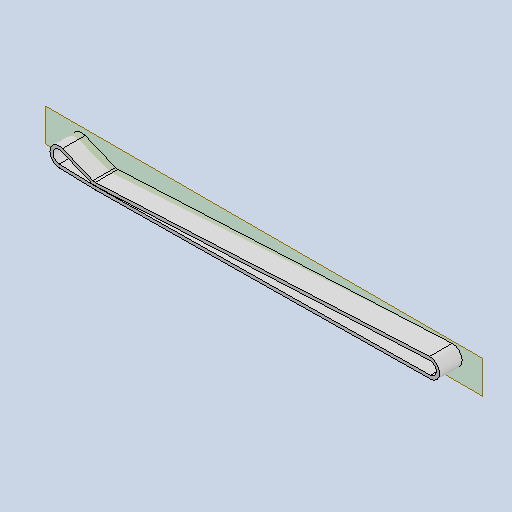
# Autodesk Inventor part: Cata rubber bands
Saved by Autodesk Inventor 2023.2 (Build 272271030, 271C)
## iProperties
Created: 2023-05-20
Part Number: Cata rubber bands
Material: Generic
Document SubType Name: Modeling
Designer: Main Account
Density: 1 g/cm^3
Appearance: Default
Author: Main Account
Autodesk Inventor part; units mm, degrees
ref_plane "YZ Plane" through (0, 0, 0) normal (1, 0, 0) x (0, 1, 0)
ref_plane "XZ Plane" through (0, 0, 0) normal (0, 1, 0) x (-1, 0, 0)
ref_plane "XY Plane" through (0, 0, 0) normal (0, 0, 1) x (1, 0, 0)
sketch "Sketch1" plane through (0, 0, 0) normal (0, 0, 1) x (1, 0, 0)
  circle A0 centre (-188.587, -221.4819) radius 3.0353 construction
  circle A1 centre (-168.9013, -220.2863) radius 3.0353 construction
  circle A2 centre (15.875, -215.9) radius 3.0353 construction
  arc A3 (-169.9939, -223.1182) -> (-168.6946, -223.3146) centre (-168.9013, -220.2863) ccw
  arc A4 (-187.3572, -218.2946) -> (-188.6171, -224.898) centre (-188.587, -221.4819) ccw
  arc A5 (-186.7273, -216.6619) -> (-188.6325, -226.648) centre (-188.587, -221.4819) ccw
  arc A6 (15.9814, -219.3146) -> (15.6425, -212.4916) centre (15.875, -215.9) ccw
  arc A7 (16.0359, -221.0638) -> (15.5233, -210.7457) centre (15.875, -215.9) ccw
  line L0 (-169.9939, -223.1182) -> (-186.7273, -216.6619)
  line L1 (-168.9589, -226.8214) -> (-188.6325, -226.648)
  line L2 (-188.6171, -224.898) -> (-168.9434, -225.0715)
  line L3 (-170.6238, -224.7509) -> (-187.3572, -218.2946)
  line L4 (-168.6946, -223.3146) -> (15.5233, -210.7457)
  line L5 (15.6425, -212.4916) -> (-168.5755, -225.0605)
  line L6 (15.9814, -219.3146) -> (-168.7523, -225.0693)
  line L7 (-168.6978, -226.8185) -> (16.0359, -221.0638)
  arc A8 (-170.6238, -224.7509) -> (-168.5755, -225.0605) centre (-168.9013, -220.2863) ccw
  arc A9 (-168.9589, -226.8214) -> (-168.6978, -226.8185) centre (-168.9013, -220.2863) ccw
  arc A10 (-164.3235, -224.9314) -> (-164.1549, -224.7589) centre (-168.9013, -220.2863) ccw
  point P0 (0, 0)
  point P1 (-192.7723, -212.6051)
  point P2 (-183.4432, -220.9999)
  point P3 (-202.7453, -212.6946)
  point P4 (-199.5727, -216.4604)
  point P5 (-186.4, -216.7421)
  dimension "d0" = 0
  dimension "d2" = 0.381
  dimension "d3" = 1.75
  dimension "d9" = 1.75
  dimension "d10" = 1.75
  dimension "d11" = 0.381
  dimension "d12" = 1.75
  constraints: 18 point on circle, 16 end point, 16 tangent, 8 centre point, 2 point on line
  measures "d0" radial gap between concentric circles of A1 A3
  measures "d2" radial gap between concentric circles of A0 A4
  measures "d3" radial gap between concentric circles of A4 A5
  measures "d9" radial gap between concentric circles of A3 A8
  measures "d10" radial gap between concentric circles of A9 A8
  measures "d11" radial gap between concentric circles of A6 A2
  measures "d12" radial gap between concentric circles of A7 A6
extrude "main bands" add sketch "Sketch1" along normal blind 12.7 and the other way blind 3.81
sketch "Sketch2" plane through (16.0359, -221.0638, -3.81) normal (0.0311361, -0.9995152, 0) x (0.9995152, 0.0311361, 0)
  line L0 (5.1663, 0) -> (5.1663, 16.51) projected
  line L1 (-184.8232, 16.51) -> (0, 16.51) projected
  line L2 (0, 0) -> (-184.8232, 0) projected
  line L3 (-209.703, 0) -> (-209.703, 16.51) projected
  line L4 (-209.703, 0) -> (-202.5278, 0) projected
  line L5 (5.1663, 4.318) -> (-209.703, 0)
  line L6 (0, 0) -> (5.1663, 0)
  line L7 (-209.703, 0) -> (-184.8232, 0)
  line L8 (-202.5278, 16.51) -> (-209.703, 16.51) projected
  line L9 (-209.703, 16.51) -> (-184.8232, 16.51)
  line L10 (5.1663, 16.51) -> (0, 16.51)
  line L11 (5.1663, 16.51) -> (-209.703, 12.192)
  point P0 (-9.145, 3.81)
  point P1 (-204.743, 0)
  point P2 (-204.743, 16.51)
  dimension "d17" = 4.318
  dimension "d18" = 4.318
  constraints: 12 end point, 2 horizontal, 2 point on line, 1 collinear, 1 parallel
  measures "d17" distance of L0.start L5.start
  measures "d18" distance of L3.end L11.end
extrude "diagonal cuts" cut sketch "Sketch2" against normal blind 25.4 contours L6 L2 L7 L4 L5 L0 | L11 L3 L8 L9 L1 L10
ref_plane "inside edge" through (0, 0, 0) normal (0, 0, -1) x (-1, 0, 0)
body "Solid1"
